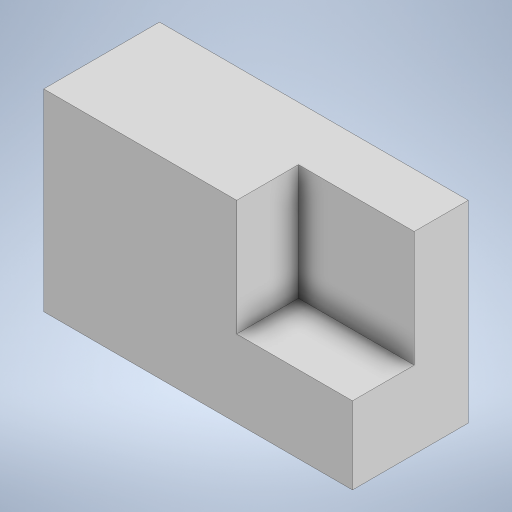
# Autodesk Inventor part: desenho 2
Saved by Autodesk Inventor 2024 (Build 280153000, 153)
## iProperties
Created: 2023-09-11
Part Number: desenho 2
Material: Generic
Document SubType Name: Modeling
Designer: LORAC
Density: 1 g/cm^3
Appearance: Default
Author: LORAC
Autodesk Inventor part; units mm, degrees
ref_plane "YZ Plane" through (0, 0, 0) normal (1, 0, 0) x (0, 1, 0)
ref_plane "XZ Plane" through (0, 0, 0) normal (0, 1, 0) x (-1, 0, 0)
ref_plane "XY Plane" through (0, 0, 0) normal (0, 0, 1) x (1, 0, 0)
sketch "Sketch1" plane through (0, 0, 0) normal (0, 0, 1) x (1, 0, 0)
  line L0 (-20, -12.5) -> (20, -12.5)
  line L1 (20, -12.5) -> (20, 12.5)
  line L2 (20, 12.5) -> (-20, 12.5)
  line L3 (-20, 12.5) -> (-20, -12.5)
  line L4 (-20, -12.5) -> (20, 12.5) construction
  line L5 (20, -12.5) -> (-20, 12.5) construction
  point P0 (0, 0)
  dimension "d0" = 40
  dimension "d1" = 25
  constraints: 12 end point, 2 midpoint, 2 parallel, 1 horizontal, 1 perpendicular
  measures "d0" distance of L2.end L1.end
  measures "d1" distance of L1.end L0.end
extrude "Extrusion1" add sketch "Sketch1" against normal blind 15
sketch "Sketch2" plane through (0, 0, 0) normal (0, 0, 1) x (1, 0, 0)
  line L0 (20, 12.5) -> (20, -12.5) projected
  line L1 (20, 12.5) -> (5, 12.5)
  line L2 (5, 12.5) -> (5, -2.5)
  line L3 (5, -2.5) -> (20, -2.5)
  line L4 (20, -2.5) -> (20, 12.5)
  point P0 (0, 0)
  dimension "d4" = 15
  dimension "d5" = 15
  constraints: 8 end point, 2 parallel, 1 horizontal, 1 perpendicular
  measures "d4" distance of L3.end L2.end
  measures "d5" distance of L2.end L1.end
extrude "Extrusion2" cut sketch "Sketch2" against normal blind 8
body "Solid1"
